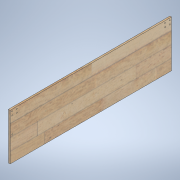
# Autodesk Inventor part: FahneHolz
Saved by Autodesk Inventor 2020.3 (Build 243373010, 373A)
## iProperties
Created: 2020-10-21
Part Number: FahneHolz
Material: Generisch
Document SubType Name: Modeling
Designer: Stefan
Density: 1 g/cm^3
Appearance: Pappel
Author: Stefan
Autodesk Inventor part; units mm, degrees
ref_plane "YZ Plane" through (0, 0, 0) normal (1, 0, 0) x (0, 1, 0)
ref_plane "XZ Plane" through (0, 0, 0) normal (0, 1, 0) x (-1, 0, 0)
ref_plane "XY Plane" through (0, 0, 0) normal (0, 0, 1) x (1, 0, 0)
sketch "Skizze1" plane through (0, 0, 0) normal (1, 0, 0) x (0, 1, 0)
  line L0 (-211.1748, 4.1838) -> (8.8252, 4.1838)
  line L1 (8.8252, 4.1838) -> (8.8252, -759.5162)
  line L2 (8.8252, -759.5162) -> (-211.1748, -759.5162)
  line L3 (-211.1748, -759.5162) -> (-211.1748, 4.1838)
  point P0 (0, 0)
  dimension "d0" = 763.7
  dimension "d1" = 220
  constraints: 8 end point, 2 parallel, 1 horizontal, 1 perpendicular
  measures "d0" distance of L0.end L1.end
  measures "d1" distance of L1.end L2.end
extrude "Extrusion1" add sketch "Skizze1" along normal blind 8
sketch "Skizze2" plane through (0, 0, 0) normal (-1, 0, 0) x (0, 0, 1)
  circle A0 centre (-4.8162, -0.1748) radius 2.5
  line L0 (4.1838, 8.8252) -> (4.1838, -211.1748) projected
  line L1 (-759.5162, 8.8252) -> (4.1838, 8.8252) projected
  circle A1 centre (-4.8162, -17.1748) radius 2.5
  circle A2 centre (-26.8162, -17.1748) radius 2.5
  circle A3 centre (-26.8162, -0.1748) radius 2.5
  line L2 (-377.7412, 9.6508) -> (-377.7412, -210.3492) construction
  line L3 (4.1838, -211.1748) -> (-759.5162, -211.1748) projected
  line L4 (-377.6662, 8.8252) -> (-157.6662, 8.8252) construction
  circle A4 centre (-750.6662, -0.1748) radius 2.5
  circle A5 centre (-750.6662, -17.1748) radius 2.5
  circle A6 centre (-728.6662, -17.1748) radius 2.5
  circle A7 centre (-728.6662, -0.1748) radius 2.5
  circle A8 centre (-6.5162, -95.6398) radius 2.5
  point P0 (0, 0)
  point P1 (-755.4823, 0)
  dimension "d4" = 5
  dimension "d5" = 9
  dimension "d6" = 9
  dimension "d7" = 5
  dimension "d8" = 5
  dimension "d9" = 5
  dimension "d10" = 17
  dimension "d11" = 9
  dimension "d12" = 22
  dimension "d13" = 17
  dimension "d14" = 17
  dimension "d15" = 22
  dimension "d17" = 381.925
  dimension "d67" = 5
  dimension "d68" = 10.7
  dimension "d69" = 104.465
  constraints: 9 centre point, 5 symmetric about line, 4 end point, 1 horizontal, 1 midpoint, 1 perpendicular, 4 other
  measures "d4" diameter of A0
  measures "d5" distance from line of L0 A0.centre
  measures "d6" distance from line of L1 A0.centre
  measures "d7" diameter of A1
  measures "d8" diameter of A2
  measures "d9" diameter of A3
  measures "d10" distance of A0.centre A1.centre
  measures "d11" distance from line of L0 A1.centre
  measures "d12" distance of A1.centre A2.centre
  measures "d13" vertical distance of A0.centre A2.centre
  measures "d14" vertical distance of A1.centre A3.centre
  measures "d15" horizontal distance of A1.centre A3.centre
  measures "d17" distance between parallel lines of L0 L2
  measures "d67" diameter of A8
  measures "d68" distance from line of L0 A8.centre
  measures "d69" distance from line of L1 A8.centre
hole "Bohrung1" at (0, -0.1748, -4.8162) direction (1, 0, 0) diameter 5 end through all
hole "Bohrung2" at (0, -17.1748, -4.8162) direction (1, 0, 0) diameter 5 end through all
hole "Bohrung3" at (0, -17.1748, -26.8162) direction (1, 0, 0) diameter 5 end through all
hole "Bohrung4" at (0, -0.1748, -26.8162) at (0, -17.1748, -750.6662) direction (1, 0, 0) diameter 5 end through all
hole "Bohrung5" at (0, -0.1748, -750.6662) direction (1, 0, 0) diameter 5 end through all
hole "Bohrung6" at (0, -0.1748, -728.6662) direction (1, 0, 0) diameter 5 end through all
hole "Bohrung7" at (0, -17.1748, -728.6662) direction (1, 0, 0) diameter 5 end through all
hole "Bohrung8" at (0, -95.6398, -6.5162) direction (1, 0, 0) diameter 5 end through all
